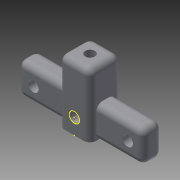
# Autodesk Inventor part: Part3
Saved by Autodesk Inventor 2015 (Build 190159000, 159)
## iProperties
Created: 2014-11-06
Part Number: Part3
Material: Generic
Document SubType Name: Modeling
Designer: ah14592
Density: 1 g/cm^3
Appearance: Default
Author: ah14592
Autodesk Inventor part; units mm, degrees
ref_plane "YZ Plane" through (0, 0, 0) normal (1, 0, 0) x (0, 1, 0)
sketch "Sketch6" plane through (0, 0, 0) normal (0, 0, 1) x (1, 0, 0)
  line L0 (-5, 5) -> (5, 5)
  line L1 (5, 5) -> (5, -5)
  line L2 (5, -5) -> (-5, -5)
  line L3 (-5, -5) -> (-5, 5)
  point P0 (0, 0)
  dimension "d31" = 10
  dimension "d32" = 10
  dimension "d33" = 5
  dimension "d34" = 5
  constraints: 8 end point, 2 parallel, 1 horizontal, 1 perpendicular
  measures "d31" distance between parallel lines of L1 L3
  measures "d32" distance between parallel lines of L2 L0
  measures "d33" distance from line of point (0, 0) L0
  measures "d34" distance from line of L3 point (0, 0)
extrude "Extrusion3" add sketch "Sketch6" along normal blind 20
sketch "Sketch7" plane through (0, 0, 20) normal (0, 0, 1) x (1, 0, 0)
  point P0 (0, 0)
  point P1 (0, 0)
  constraints: 1 coincident
hole "Hole4" at (0, 0, 20) direction (0, 0, -1) diameter 3.1 depth 8
sketch "Sketch8" plane through (-5, 5, 0) normal (0, 1, 0) x (1, 0, 0)
  point P0 (5, 0)
  point P1 (5, -5)
  dimension "d44" = 5
  measures "d44" distance of point (5, -5) point (5, 0)
hole "Hole5" at (0, 5, 5) direction (0, -1, 0) diameter 3.3 end through all counterbore diameter 4.1 counterbore depth 5
sketch "Sketch9" plane through (5, -5, 0) normal (1, 0, 0) x (0, 0, -1)
  line L0 (0, 10) -> (-20, 10) construction
  line L1 (-10, 10) -> (-10, 0) construction
  line L2 (0, 0) -> (-20, 0) construction
  line L3 (0, 0) -> (0, 10) projected
  line L4 (-10, 8) -> (0, 8)
  line L5 (0, 8) -> (0, 2)
  line L6 (0, 2) -> (-10, 2)
  line L7 (-10, 2) -> (-10, 8)
  line L8 (0, 5) -> (-20, 5)
  line L9 (-20, 10) -> (-20, 0) projected
  dimension "d52" = 6
  constraints: 12 end point, 3 midpoint, 2 parallel, 2 point on line, 1 horizontal, 1 perpendicular, 1 other
  measures "d52" distance between parallel lines of L6 L4
extrude "Extrusion4" add sketch "Sketch9" along normal blind 15
ref_plane "Work Plane2" through (5, 3, 2) normal (0, 1, 0) x (1, 0, 0)
ref_plane "Work Plane1" through (0, -3, 18) normal (1, 0, 0) x (0, 0, -1)
mirror "Mirror1" about plane through (0, -3, 18) normal (1, 0, 0) of "Extrusion4"
fillet "Fillet3" radius 2 6 edges at (-12.5, 3, 0) (-12.5, 3, 10) (12.5, 3, 10) (-12.5, -3, 10) (12.5, -3, 10) (-12.5, -3, 0)
fillet "Fillet4" radius 2 10 edges at (12.5, 3, 0) (12.5, -3, 0) (5, 5, 10) (-5, 5, 10) (-5, -5, 10) (5, -5, 10) (-5, 0, 20) (5, 0, 20) (0, 5, 20) (0, -5, 20)
fillet "Fillet5" radius 2 14 edges at (20, -2.4144, 0.5856) (20, -3, 4.9997) (20, 0, 0) (20, 2.4144, 0.5856) (20, 3, 4.9997) (20, 0, 10) (-20, 0, 10) (-20, -2.4142, 9.4142) (-20, -3, 5) (-20, -2.4142, 0.5858) (-20, 0, 0) (-20, 2.4142, 0.5858) (-20, 3, 5) (-20, 2.4142, 9.4142)
sketch "Sketch11" plane through (-3, -5, 0) normal (0, -1, 0) x (1, 0, 0)
  circle A0 centre (3, 5) radius 1.65 projected
  point P0 (3, 0)
  constraints: 1 coincident
sketch "Sketch12" plane through (5, 3, 8) normal (0, 1, 0) x (1, 0, 0)
  line L0 (0, 6) -> (0, 0) construction
  line L1 (0, 3) -> (15, 3) construction
  line L2 (15, 0) -> (15, 6) construction
  line L3 (-10, 0) -> (-10, 6) construction
  line L4 (-10, 3) -> (-25, 3) construction
  line L5 (-25, 6) -> (-25, 0) construction
  point P0 (-5, 8)
  point P1 (10, 3)
  point P2 (-20, 3)
  dimension "d67" = 5
  dimension "d68" = 5
  constraints: 4 end point, 4 midpoint, 2 point on line
  measures "d67" distance from line of L2 point (10, 3)
  measures "d68" distance from line of L5 point (-20, 3)
hole "Hole7" at (15, 3, 5) at (-15, 3, 5) direction (0, -1, 0) diameter 3.3 end through all counterbore diameter 4.1 counterbore depth 4
body "Solid2"
